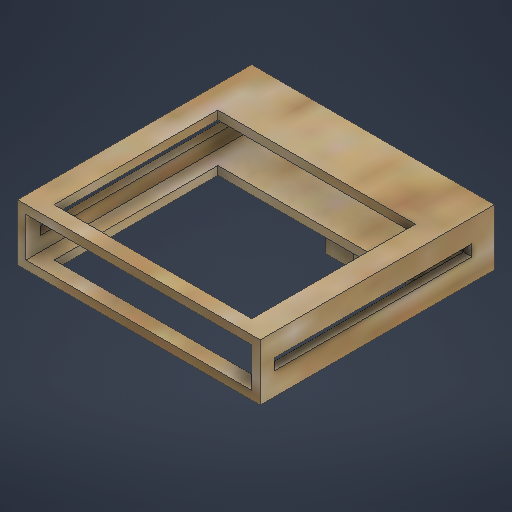
# Autodesk Inventor part: shot_glass_tray
Saved by Autodesk Inventor 2026.1 (Build 301233000, 233)
## iProperties
Created: 2025-10-10
Part Number: shot_glass_tray
Material: Generic
Document SubType Name: Modeling
Designer: Ethan
Density: 1 g/cm^3
Appearance: Plywood - Weathered
Author: Ethan
Autodesk Inventor part; units mm, degrees
ref_plane "YZ Plane" through (0, 0, 0) normal (1, 0, 0) x (0, 1, 0)
ref_plane "XZ Plane" through (0, 0, 0) normal (0, 1, 0) x (-1, 0, 0)
ref_plane "XY Plane" through (0, 0, 0) normal (0, 0, 1) x (1, 0, 0)
sketch "Sketch1" plane through (0, 0, 0) normal (0, 0, 1) x (1, 0, 0)
  line L0 (0, 0) -> (-9.9, 0)
  line L1 (-9.9, 0) -> (-9.9, 10)
  line L2 (-9.9, 10) -> (0, 10)
  line L3 (0, 10) -> (0, 0)
  dimension "d0" = 9.9
  dimension "d1" = 10
  constraints: 8 end point, 2 parallel, 1 horizontal, 1 perpendicular
  measures "d0" distance of L1.end L2.end
  measures "d1" distance of L0.end L1.end
extrude "Extrusion1" add sketch "Sketch1" along normal blind 9.9
sketch "Sketch2" plane through (0, 0, 0) normal (1, 0, 0) x (0, 0, -1)
  circle A0 centre (-5, 5) radius 2
  line L0 (0, 0) -> (-9.9, 0) projected
  line L1 (0, 0) -> (0, 10) projected
  point P0 (-4.95, 0)
  dimension "d4" = 4
  dimension "d5" = 5
  dimension "d6" = 5
  constraints: 1 centre point, 1 midpoint
  measures "d4" diameter of A0
  measures "d5" vertical distance of point (-4.95, 0) A0.centre
  measures "d6" distance from line of L1 A0.centre
extrude "Extrusion2" cut sketch "Sketch2" against normal blind 10
sketch "Sketch3" plane through (-9.9, 10, 0) normal (0, 1, 0) x (1, 0, 0)
  line L0 (0, 0) -> (0, -9.9) projected
  circle A0 centre (4.95, -4.95) radius 7.0004
  line L1 (9.9, 0) -> (0, 0) projected
  line L2 (-2.0504, -11.9504) -> (11.9504, -11.9504)
  line L3 (11.9504, -11.9504) -> (11.9504, 2.0504)
  line L4 (11.9504, 2.0504) -> (-2.0504, 2.0504)
  line L5 (-2.0504, 2.0504) -> (-2.0504, -11.9504)
  point P0 (-2.0504, -4.95)
  point P1 (4.95, 2.0504)
  point P2 (4.95, -11.9504)
  point P3 (11.9504, -4.95)
  dimension "d9" = 4.95
  dimension "d10" = 4.95
  constraints: 8 end point, 2 parallel, 1 horizontal, 1 perpendicular, 3 other
  measures "d9" distance from line of point (4.95, -4.95) L1
  measures "d10" distance from line of L0 point (4.95, -4.95)
extrude "Extrusion3" add sketch "Sketch3" along normal blind 3
sketch "Sketch14" plane through (-9.9, 13, 0) normal (0, 1, 0) x (1, 0, 0)
  line L0 (-35.05, -80.9496) -> (44.95, -80.9496)
  line L1 (44.95, -80.9496) -> (44.95, 2.0504)
  line L2 (44.95, 2.0504) -> (-35.05, 2.0504)
  line L3 (-35.05, 2.0504) -> (-35.05, -80.9496)
  line L4 (11.9504, 2.0504) -> (-2.0504, 2.0504) projected
  line L5 (-35.05, 2.0504) -> (-38.05, 2.0504)
  line L6 (-38.05, 2.0504) -> (-38.05, -80.9496)
  line L7 (-38.05, -80.9496) -> (-35.05, -80.9496)
  line L8 (-35.05, -80.9496) -> (-35.05, 2.0504)
  line L9 (44.95, -80.9496) -> (47.95, -80.9496)
  line L10 (47.95, -80.9496) -> (47.95, 2.0504)
  line L11 (47.95, 2.0504) -> (44.95, 2.0504)
  line L12 (44.95, 2.0504) -> (44.95, -80.9496)
  point P0 (9.9, 0)
  point P1 (-35.05, -39.4496)
  point P2 (4.95, 2.0504)
  point P3 (4.95, 2.0504)
  point P4 (44.95, 2.0504)
  dimension "d60" = 40
  dimension "d61" = 40
  dimension "d62" = 0
  dimension "d63" = 83
  dimension "d64" = 3
  dimension "d65" = 3
  dimension "d68" = 83
  constraints: 24 end point, 6 parallel, 3 horizontal, 3 midpoint, 3 perpendicular
  measures "d60" horizontal distance of point (-35.05, -39.45) point (4.95, 2.05)
  measures "d61" distance from line of point (4.95, 2.05) L1
  measures "d62" distance between parallel lines of L4 L2
  measures "d63" distance of L2.end L0.start
  measures "d64" distance of L7.end L6.end
  measures "d65" distance of L11.end L10.end
  measures "d68" distance of L5.end L6.end
extrude "Extrusion14" add sketch "Sketch14" along normal blind 3
sketch "Sketch15" plane through (-9.9, 16, 0) normal (0, 1, 0) x (1, 0, 0)
  line L0 (-2.0504, 2.0504) -> (-38.05, 2.0504) projected
  line L1 (-38.05, -80.9496) -> (47.95, -80.9496) projected
  line L2 (-38.05, 2.0504) -> (-35.05, 2.0504)
  line L3 (-35.05, 2.0504) -> (-35.05, -80.9496)
  line L4 (-35.05, -80.9496) -> (-38.05, -80.9496)
  line L5 (-38.05, -80.9496) -> (-38.05, 2.0504)
  line L6 (47.95, -80.9496) -> (47.95, 2.0504) projected
  line L7 (47.95, 2.0504) -> (44.95, 2.0504)
  line L8 (44.95, 2.0504) -> (44.95, -80.9496)
  line L9 (44.95, -80.9496) -> (47.95, -80.9496)
  line L10 (47.95, -80.9496) -> (47.95, 2.0504)
  line L11 (-38.05, 2.0504) -> (47.95, 2.0504)
  line L12 (47.95, 2.0504) -> (47.95, -0.9496)
  line L13 (47.95, -0.9496) -> (-38.05, -0.9496)
  line L14 (-38.05, -0.9496) -> (-38.05, 2.0504)
  point P0 (9.9, 0)
  point P1 (-35.05, -0.9496)
  point P2 (44.95, -0.9496)
  dimension "d69" = 3
  dimension "d70" = 3
  dimension "d71" = 3
  constraints: 24 end point, 6 parallel, 3 horizontal, 3 perpendicular, 3 point on line
  measures "d69" distance of L3.end L4.end
  measures "d70" distance of L9.end L8.end
  measures "d71" distance between parallel lines of L11 L13
extrude "Extrusion15" add sketch "Sketch15" along normal blind 14 contours L11 L8 L13 L3 L0 | L3 L13 L5 L0 | L7 L6 L13 L8 | L3 L1 L5 L13 | L13 L6 L1 L8
sketch "Sketch16" plane through (-9.9, 30, 0) normal (0, 1, 0) x (1, 0, 0)
  line L0 (47.95, 2.0504) -> (-38.05, 2.0504) projected
  line L1 (47.95, -80.9496) -> (47.95, 2.0504) projected
  line L2 (-38.05, 2.0504) -> (47.95, 2.0504)
  line L3 (47.95, 2.0504) -> (47.95, -80.9496)
  line L4 (47.95, -80.9496) -> (-38.05, -80.9496)
  line L5 (-38.05, -80.9496) -> (-38.05, 2.0504)
  point P0 (9.9, 0)
  constraints: 8 end point, 2 parallel, 1 horizontal, 1 perpendicular
extrude "Extrusion16" add sketch "Sketch16" along normal blind 3
sketch "Sketch17" plane through (-9.9, 13, 0) normal (0, -1, 0) x (1, 0, 0)
  line L0 (39.95, 75.9496) -> (-30.05, 75.9496)
  line L1 (-30.05, 75.9496) -> (-30.05, 17.9496)
  line L2 (-30.05, 17.9496) -> (39.95, 17.9496)
  line L3 (39.95, 17.9496) -> (39.95, 75.9496)
  line L4 (47.95, -2.0504) -> (11.9504, -2.0504) projected
  line L5 (44.95, 80.9496) -> (44.95, 0.9496) projected
  line L6 (-38.05, 80.9496) -> (47.95, 80.9496) projected
  line L7 (-35.05, 0.9496) -> (-35.05, 80.9496) projected
  point P0 (9.9, 0)
  dimension "d76" = 20
  dimension "d77" = 5
  dimension "d78" = 5
  dimension "d79" = 5
  constraints: 8 end point, 2 parallel, 1 horizontal, 1 perpendicular
  measures "d76" distance between parallel lines of L4 L2
  measures "d77" distance between parallel lines of L5 L3
  measures "d78" distance between parallel lines of L6 L0
  measures "d79" distance between parallel lines of L7 L1
extrude "Extrusion17" cut sketch "Sketch17" against normal blind 33
sketch "Sketch18" plane through (38.05, 13, 80.9496) normal (1, 0, 0) x (0, 0, -1)
  line L0 (5, 12) -> (75, 12)
  line L1 (75, 12) -> (75, 8)
  line L2 (75, 8) -> (5, 8)
  line L3 (5, 8) -> (5, 12)
  line L4 (80, 17) -> (0, 17) projected
  line L5 (0, 3) -> (80, 3) projected
  line L6 (80, 3) -> (80, 17) projected
  line L7 (0, 0) -> (0, 20) projected
  point P0 (80.9496, -13)
  point P1 (80, 10)
  point P2 (75, 10)
  point P3 (0, 10)
  point P4 (5, 10)
  dimension "d82" = 5
  dimension "d83" = 5
  dimension "d84" = 5
  dimension "d85" = 5
  constraints: 8 end point, 4 midpoint, 2 parallel, 1 horizontal, 1 perpendicular
  measures "d82" distance between parallel lines of L4 L0
  measures "d83" distance between parallel lines of L5 L2
  measures "d84" distance of point (80, 10) point (75, 10)
  measures "d85" distance of point (0, 10) point (5, 10)
extrude "Extrusion18" cut sketch "Sketch18" against normal blind 333 contours L0 L1 L2 L3
body "Solid1"
